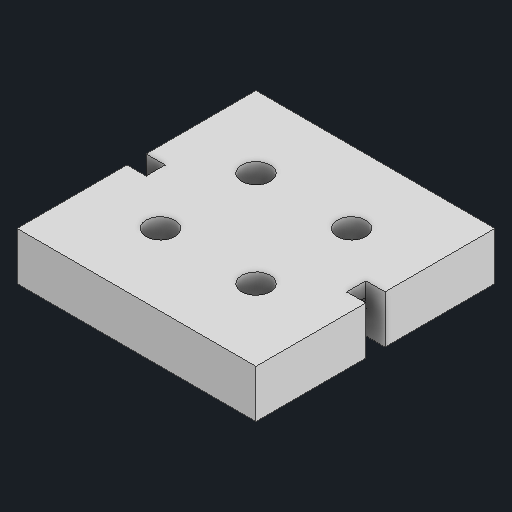
# Autodesk Inventor part: 2_inner_leg_top_plate
Saved by Autodesk Inventor 2024 (Build 280153000, 153)
## iProperties
Created: 2023-05-23
Part Number: 2_inner_leg_top_plate
Material: Generic
Document SubType Name: Modeling
Designer: aasmu
Density: 1 g/cm^3
Appearance: Default
Author: aasmu
Autodesk Inventor part; units mm, degrees
ref_plane "YZ Plane" through (0, 0, 0) normal (1, 0, 0) x (0, 1, 0)
ref_plane "XZ Plane" through (0, 0, 0) normal (0, 1, 0) x (-1, 0, 0)
ref_plane "XY Plane" through (0, 0, 0) normal (0, 0, 1) x (1, 0, 0)
sketch "Sketch2" plane through (0, 0, 0) normal (0, 1, 0) x (-1, 0, 0)
  line L0 (0, 0) -> (-50, 0)
  line L1 (-50, 0) -> (-50, -50)
  line L2 (-50, -50) -> (0, -50)
  line L3 (0, -50) -> (0, 0)
  circle A0 centre (-15, -35) radius 3
  circle A1 centre (-15, -15) radius 3
  line L4 (-15, -35) -> (-15, -50) construction
  line L5 (-15, -15) -> (-15, 0)
  line L6 (-15, -35) -> (0, -35) construction
  line L7 (0, -27) -> (-4, -27)
  line L8 (-4, -23) -> (0, -23)
  line L9 (0, -23) -> (0, -27)
  line L10 (-50, -27) -> (-46, -27)
  line L11 (-46, -23) -> (-50, -23)
  line L12 (-50, -23) -> (-50, -27)
  line L13 (-50, -30) -> (-50, -37)
  line L14 (0, -13) -> (0, -20)
  line L15 (-4, -23) -> (-4, -19)
  line L16 (-4, -19) -> (-46, -19)
  line L17 (-46, -19) -> (-46, -23)
  line L18 (-46, -27) -> (-46, -31)
  line L19 (-46, -31) -> (-4, -31)
  line L20 (-4, -31) -> (-4, -27)
  line L21 (-4, -27) -> (-4, -23)
  line L22 (-46, -27) -> (-46, -23)
  line L23 (-35, 0) -> (-35, -15) construction
  line L24 (-35, -50) -> (-35, -35) construction
  line L25 (-35, -15) -> (-50, -15) construction
  circle A2 centre (-35, -15) radius 3
  circle A3 centre (-35, -35) radius 3
  point P0 (0, -25)
  point P1 (-50, -25)
  point P2 (0, -23)
  dimension "d0" = 50
  dimension "d1" = 6
  dimension "d6" = 4
  dimension "d10" = 7
  dimension "d23" = 15
  dimension "d24" = 4
  constraints: 52 end point, 18 equal length, 8 point on line, 7 perpendicular, 7 vertical, 4 centre point, 4 horizontal, 3 equal radius, 2 coincident, 2 collinear, 2 midpoint
  measures "d0" distance of L2.end L0.start
  measures "d1" diameter of A0
  measures "d6" distance of L7.end L8.start
  measures "d10" distance of L13.start L13.end
  measures "d23" distance of L4.start L4.end
  measures "d24" distance of L10.end L18.end
extrude "Extrusion1" add sketch "Sketch2" along normal blind 10 contours L3 L8 L15 L16 L17 L11 L1 L0 | L10 L18 L19 L20 L7 L3 L2 L1 | L17 L16 L15 L21 L20 L19 L18 L22
extrude "Extrusion2" cut sketch "Sketch2" along normal blind 5 contours L17 L16 L15 L21 L20 L19 L18 L22
fillet "Fillet1" radius 2 2 edges at (4, 5, -25) (46, 5, -25)
equation "\"d0\" = width"
equation "\"d1\" = hole_diameter"
equation "\"d6\" = cabel_shaft_size"
equation "\"d23\" = edge_to_hole"
equation "\"d24\" = cabel_shaft_size"
equation "\"d18\" = plate_thicknes"
equation "\"d20\" = 0.5 * plate_thicknes"
equation "\"width\" = inner_leg_width"
equation "\"cabel_channel_depth\" = 4"
equation "\"plate_thicknes\" = 10"
equation "\"hole_diameter\" = 6"
equation "\"cabel_shaft_size\" = 4"
equation "\"edge_to_hole\" = 15"
equation "\"inner_leg_width\" = 50"
body "Solid1"
